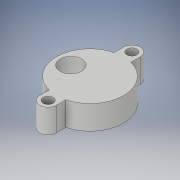
# Autodesk Inventor part: footprint
Saved by Autodesk Inventor 2019 (Build 230136000, 136)
## iProperties
Created: 2019-04-09
Part Number: footprint
Material: Generic
Document SubType Name: Modeling
Designer: jmc
Density: 1 g/cm^3
Appearance: Default
Author: jmc
Autodesk Inventor part; units mm, degrees
ref_plane "YZ Plane" through (0, 0, 0) normal (1, 0, 0) x (0, 1, 0)
ref_plane "XZ Plane" through (0, 0, 0) normal (0, 1, 0) x (-1, 0, 0)
ref_plane "XY Plane" through (0, 0, 0) normal (0, 0, 1) x (1, 0, 0)
sketch "Sketch1" plane through (0, 0, 0) normal (0, 1, 0) x (-1, 0, 0)
  line L0 (0, 17.5) -> (0, -17.5) construction
  circle A0 centre (0, 17.5) radius 2.1
  circle A1 centre (0, -17.5) radius 2.1
  line L1 (0, 0) -> (8, 0) construction
  circle A2 centre (8, 0) radius 4.5
  arc A3 (3.5, 17.5) -> (-3.5, 17.5) centre (0, 17.5) ccw
  arc A4 (-3.5, -17.5) -> (3.5, -17.5) centre (0, -17.5) ccw
  line L2 (3.5, 17.5) -> (3.5, 13.5554)
  line L3 (-3.5, 17.5) -> (-3.5, 13.5554)
  line L4 (3.5, -17.5) -> (3.5, -13.5554)
  line L5 (-3.5, -17.5) -> (-3.5, -13.5554)
  arc A5 (3.5, -13.5554) -> (3.5, 13.5554) centre (0, 0) ccw
  arc A6 (-3.5, 13.5554) -> (-3.5, -13.5554) centre (0, 0) ccw
  dimension "d0" = 35
  dimension "d1" = 4.2
  dimension "d2" = 4.2
  dimension "d3" = 8
  dimension "d4" = 9
  dimension "d8" = 7
  dimension "d9" = 7
  constraints: 12 end point, 8 point on circle, 7 centre point, 5 coincident, 4 point on line, 2 tangent, 2 vertical, 1 horizontal, 1 midpoint, 1 parallel
  measures "d0" distance of L0.start L0.end
  measures "d1" diameter of A0
  measures "d2" diameter of A1
  measures "d3" distance of L1.start L1.end
  measures "d4" diameter of A2
  measures "d8" diameter of A4
  measures "d9" diameter of A3
extrude "Extrusion1" add sketch "Sketch1" along normal blind 10
body "Solid1"
